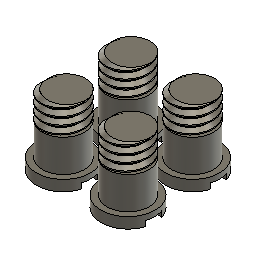
MyPad (Autodesk Fusion 360 archive; units mm, degrees)
design "Screws"
Autodesk Fusion 360 part; units mm, degrees
sketch "Sketch1" plane through (0, 0, 0) normal (0, 1, 0) x (1, 0, 0)
  circle A0 centre (0, 0) radius 2.5
  circle A1 centre (0, 0) radius 2
  dimension "d1" = 5
  dimension "d2" = 4
  constraint coincident A0.centre A1.centre
  measures "d1" diameter of A0
  measures "d2" diameter of A1
extrude "Extrude1" add sketch "Sketch1" along normal blind 1 contours A0 | A1 makes body 1
extrude "Extrude2" add sketch "Sketch1" along normal blind 6.5 contours A1 bodies 1
thread "Thread1" "ISO Metric profile 4.0 M4x0.7 M4x0.7 6g" major diameter 3.908 minor diameter 3.111 pitch 0.7 angle 60 modelled right hand crest width 0.1017 on face at (1.9901, 2.8333, -0.1991) from (0, 4, 0) to (0, 6.5, 0) crest through (1.954, 0.825, 0) on bodies 1
sketch "Sketch2" plane through (0, 0, 0) normal (0, 1, 0) x (1, 0, 0)
  line L0 (2.5168, -0.75) -> (-2.5168, -0.75)
  line L1 (-2.5168, -0.75) -> (-2.5168, 0.75)
  line L2 (-2.5168, 0.75) -> (2.5168, 0.75)
  line L3 (2.5168, 0.75) -> (2.5168, -0.75)
  line L4 (2.5168, -0.75) -> (-2.5168, 0.75) construction
  line L5 (-2.5168, -0.75) -> (2.5168, 0.75) construction
  dimension "d9" = 1.5
  constraint horizontal L0
  constraint perpendicular L0 L1
  constraint parallel L0 L2
  constraint parallel L1 L3
  constraint coincident L4 origin
  constraint coincident L5 origin
  measures "d9" distance of L0.end L1.end
extrude "Extrude5" cut sketch "Sketch2" along normal blind 0.5 bodies 1
copy_body "CopyPasteBodies5" bodies 1 makes body 2
move_body "Move5" bodies 2 to x (1, 0, 0) y (0, 1, 0) z (0, 0, 1) at (6, 0, 0)
copy_body "CopyPasteBodies6" bodies 1 2 makes body 3 makes body 4
move_body "Move6" bodies 3 4 to x (1, 0, 0) y (0, 1, 0) z (0, 0, 1) at (0, 0, -6)
